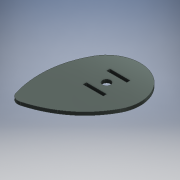
# Autodesk Inventor part: leva00
Saved by Autodesk Inventor 2016 (Build 200138000, 138)
## iProperties
Created: 2016-09-20
Part Number: leva00
Material: Madera (abedul)
Document SubType Name: Modeling
Designer: i95sa
Density: 0.55 g/cm^3
Appearance: Gris plomo - Pulido
Author: i95sa
Autodesk Inventor part; units mm, degrees
ref_plane "YZ Plane" through (0, 0, 0) normal (1, 0, 0) x (0, 1, 0)
ref_plane "XZ Plane" through (0, 0, 0) normal (0, 1, 0) x (-1, 0, 0)
ref_plane "XY Plane" through (0, 0, 0) normal (0, 0, 1) x (1, 0, 0)
sketch "Boceto1" plane through (0, 0, 0) normal (0, 0, 1) x (1, 0, 0)
  arc A0 (20.1349, 36.6252) -> (-20.1349, -36.6252) centre (0, 0) ccw
  arc A1 (-30.986, -56.3634) -> (-40.279, -73.2673) centre (-35.6325, -64.8153) ccw
  line L0 (-41.6243, -75.7144) -> (-50.0763, -71.0679)
  line L1 (-36.3842, 20.5673) -> (-50.4708, 28.3115)
  line L2 (-50.4708, 28.3115) -> (-50.0763, -71.0679)
  line L3 (-50.0763, -71.0679) -> (-50.2294, -32.4882)
  arc A2 (-36.3842, 20.5673) -> (-50.2294, -32.4882) centre (56.7214, -32.0636) ccw
  arc A3 (-50.2294, -32.4882) -> (-44.8477, -67.6627) centre (70.5423, -32.0088) ccw
  line L4 (1.5488, 2.8173) -> (20.1349, 36.6252)
  line L5 (-1.5488, -2.8173) -> (-41.6243, -75.7144)
  arc A4 (-20.1349, -36.6252) -> (20.1349, 36.6252) centre (0, 0) ccw
  arc A5 (-40.279, -73.2673) -> (-30.986, -56.3634) centre (-35.6325, -64.8153) ccw
  line L6 (-41.6243, -75.7144) -> (-33.1724, -80.3609)
  line L7 (36.8612, -19.6996) -> (50.9478, -27.4438)
  line L8 (50.9478, -27.4438) -> (-33.1724, -80.3609)
  line L9 (-33.1724, -80.3609) -> (-0.5164, -59.8182)
  arc A6 (-0.5164, -59.8182) -> (36.8612, -19.6996) centre (-57.4651, 30.7109) ccw
  arc A7 (-33.0989, -74.1216) -> (-0.5164, -59.8182) centre (-64.8243, 42.4096) ccw
  dimension "d0" = 83.59
  dimension "d6" = 19.29
  dimension "d7" = 9.645
  dimension "d8" = 16.075
  dimension "d9" = 38.58
  constraints: 20 end point, 20 point on circle, 8 centre point, 6 symmetric about line, 5 point on line, 4 tangent, 1 collinear, 4 other
  measures "d0" diameter of A0
  measures "d6" diameter of A1
  measures "d7" distance of L0.start L0.end
  measures "d8" distance of L1.start L1.end
  measures "d9" distance of L0.end L3.end
extrude "Extrusión2" add sketch "Boceto1" along normal blind 4 contours A4 A0 | A0 L5 A1 A3 A2 | A6 A7 A5 L5 A4 | L5 A1 | A5 L5
sketch "Boceto2" plane through (0, 0, 4) normal (0, 0, 1) x (1, 0, 0)
  line L0 (0, 0) -> (0, 12.5)
  line L1 (0, 12.5) -> (-12.5, 12.5)
  line L2 (-12.5, 12.5) -> (-12.5, 16.7)
  line L3 (-12.5, 16.7) -> (12.5, 16.7)
  line L4 (12.5, 16.7) -> (12.5, 12.5)
  line L5 (12.5, 12.5) -> (0, 12.5)
  line L6 (0, 0) -> (12.5, 0)
  line L7 (0, 0) -> (0, -12.5)
  line L8 (0, -12.5) -> (-12.5, -12.5)
  line L9 (-12.5, -12.5) -> (-12.5, -16.7)
  line L10 (-12.5, -16.7) -> (12.5, -16.7)
  line L11 (12.5, -16.7) -> (12.5, -12.5)
  line L12 (12.5, -12.5) -> (0, -12.5)
  circle A0 centre (0, 0) radius 5
  dimension "d24" = 12.5
  dimension "d25" = 12.5
  dimension "d26" = 4.2
  dimension "d27" = 25
  dimension "d28" = 10
  constraints: 26 end point, 5 perpendicular, 5 symmetric about line, 3 point on line, 1 centre point, 1 coincident, 1 parallel, 1 vertical
  measures "d24" distance of L0.start L0.end
  measures "d25" distance of L0.end L1.end
  measures "d26" distance of L1.end L2.end
  measures "d27" distance of L2.end L3.end
  measures "d28" diameter of A0
extrude "Extrusión3" cut sketch "Boceto2" against normal blind 4
